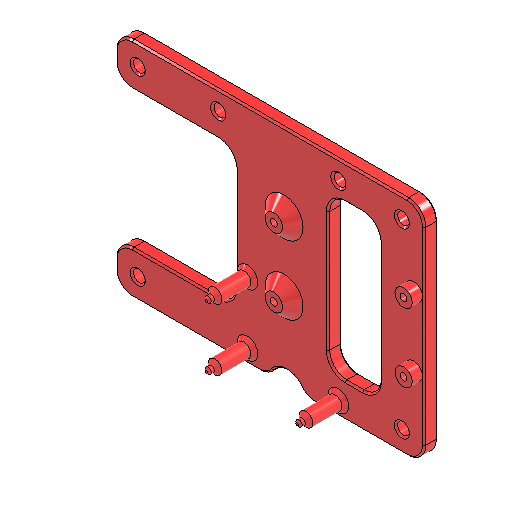
# Autodesk Inventor part: temp-logger-shelf
Saved by Autodesk Inventor 2026 (Build 300175050, 175E)
## iProperties
Created: 2025-07-16
Part Number: temp-logger-shelf
Material: ABS Plastic
Document SubType Name: Modeling
Designer: kuzmin
Density: 1.06 g/cm^3
Appearance: Light Red
Author: kuzmin
Autodesk Inventor part; units mm, degrees
ref_plane "YZ Plane" through (0, 0, 0) normal (1, 0, 0) x (0, 1, 0)
ref_plane "XZ Plane" through (0, 0, 0) normal (0, 1, 0) x (-1, 0, 0)
ref_plane "XY Plane" through (0, 0, 0) normal (0, 0, 1) x (1, 0, 0)
sketch "Sketch1" plane through (0, 0, 0) normal (0, 0, 1) x (1, 0, 0)
  line L0 (-45, 32.5) -> (45, 32.5)
  line L1 (45, 32.5) -> (45, -32.5)
  line L2 (45, -32.5) -> (-45, -32.5)
  line L3 (-45, -32.5) -> (-45, 32.5)
  line L4 (-38.5, 26.5) -> (38.5, 26.5) construction
  line L5 (38.5, 26.5) -> (38.5, -26.5) construction
  line L6 (38.5, -26.5) -> (-38.5, -26.5) construction
  line L7 (-38.5, -26.5) -> (-38.5, 26.5) construction
  circle A0 centre (-38.5, 26.5) radius 2
  circle A1 centre (38.5, 26.5) radius 2
  circle A2 centre (38.5, -26.5) radius 2
  circle A3 centre (-38.5, -26.5) radius 2
  point P0 (0, 0)
  point P1 (45, 0)
  point P2 (0, 32.5)
  point P3 (38.5, 0)
  point P4 (0, 26.5)
  dimension "d0" = 90
  dimension "d1" = 65
  dimension "d2" = 77
  dimension "d3" = 53
  dimension "d14" = 4
  constraints: 16 end point, 8 coincident, 4 centre point, 4 midpoint, 4 parallel, 3 equal radius, 2 horizontal, 2 horizontal alignment, 2 perpendicular, 2 vertical alignment
  measures "d0" distance of L0.start L0.end
  measures "d1" distance of L0.end L1.end
  measures "d2" distance of L4.start L4.end
  measures "d3" distance of L4.end L5.end
  measures "d14" diameter of A0
extrude "Extrusion1" add sketch "Sketch1" along normal blind 4 contours L0 L1 L2 L3 | A0 | A1 | A2 | A3
hole "Hole1" at (38.5, 26.5, 0) at (38.5, -26.5, 0) at (-38.5, -26.5, 0) at (-38.5, 26.5, 0) direction (0, 0, 1) diameter 3.4 end through all
sketch "Sketch2" plane through (0, 0, 4) normal (0, 0, 1) x (1, 0, 0)
  line L0 (-45, 20) -> (-10, 20)
  line L1 (-10, 20) -> (-10, -20)
  line L2 (-10, -20) -> (-45, -20)
  line L3 (-45, -20) -> (-45, 20)
  line L4 (-45, 32.5) -> (-45, -32.5) projected
  point P0 (0, 0)
  point P1 (-10, 0)
  dimension "d23" = 40
  dimension "d24" = 35
  constraints: 8 end point, 2 parallel, 1 horizontal, 1 horizontal alignment, 1 midpoint, 1 perpendicular, 1 point on line
  measures "d23" distance of L2.end L0.start
  measures "d24" distance of L0.start L0.end
extrude "Extrusion3" cut sketch "Sketch2" against normal blind 10
sketch "Sketch3" plane through (0, 0, 0) normal (0, 0, -1) x (-1, 0, 0)
  line L0 (-42, 10) -> (-4.2, 10) construction
  line L1 (-4.2, 10) -> (-4.2, -10) construction
  line L2 (-4.2, -10) -> (-42, -10) construction
  line L3 (-42, -10) -> (-42, 10) construction
  circle A0 centre (-42, 10) radius 2.5
  circle A1 centre (-4.2, 10) radius 2.5
  circle A2 centre (-4.2, -10) radius 2.5
  circle A3 centre (-42, -10) radius 2.5
  line L4 (-40, -32.5) -> (40, -32.5) projected
  line L5 (-45, -32.5) -> (-45, 32.5) projected
  point P0 (0, 0)
  point P1 (-4.2, 0)
  point P2 (-45, -27.5)
  point P3 (-45, 27.5)
  dimension "d27" = 20
  dimension "d28" = 37.8
  dimension "d30" = 5
  dimension "d47" = 3
  constraints: 8 coincident, 8 end point, 4 centre point, 3 equal radius, 2 parallel, 1 horizontal, 1 horizontal alignment, 1 midpoint, 1 perpendicular
  measures "d27" distance of L0.end L1.end
  measures "d28" distance of L0.start L0.end
  measures "d30" diameter of A1
  measures "d47" distance between parallel lines of L5 L3
extrude "Extrusion4" add sketch "Sketch3" against normal blind 7
hole "Hole2" at (4.2, 10, 0) at (4.2, -10, 0) at (42, -10, 0) at (42, 10, 0) direction (0, 0, 1) diameter 2 end through all
chamfer "Chamfer3" distance 3 angle 45 2 edges at (6.7, 10, 4) (6.7, -10, 4)
sketch "Sketch4" plane through (0, 0, 4) normal (0, 0, 1) x (1, 0, 0)
  line L0 (17, -22.5) -> (32, -22.5)
  line L1 (32, -22.5) -> (32, 22.5)
  line L2 (32, 22.5) -> (17, 22.5)
  line L3 (17, 22.5) -> (17, -22.5)
  line L4 (45, -32.5) -> (45, 32.5) projected
  line L5 (-45, -32.5) -> (45, -32.5) projected
  line L6 (0, -32.5) -> (10, -32.5)
  line L7 (10, -32.5) -> (10, -28.5)
  line L8 (10, -28.5) -> (0, -28.5)
  line L9 (0, -28.5) -> (0, -32.5)
  line L10 (-10, 20) -> (-10, -20) projected
  point P0 (0, 0)
  point P1 (17, 0)
  point P2 (45, -27.5)
  point P3 (45, 27.5)
  point P4 (-40, -32.5)
  point P5 (40, -32.5)
  point P6 (-10, 15)
  point P7 (-10, -15)
  dimension "d48" = 15
  dimension "d49" = 13
  dimension "d50" = 45
  dimension "d51" = 10
  dimension "d52" = 10
  dimension "d53" = 4
  constraints: 16 end point, 4 parallel, 2 horizontal, 2 midpoint, 2 perpendicular, 1 horizontal alignment
  measures "d48" distance of L1.end L2.end
  measures "d49" distance between parallel lines of L4 L1
  measures "d50" distance of L2.end L0.start
  measures "d51" distance between parallel lines of L10 L9
  measures "d52" distance of L7.end L8.end
  measures "d53" distance of L6.end L7.end
extrude "Extrusion5" cut sketch "Sketch4" against normal through all
fillet "Fillet2" radius 5 16 edges at (-10, -20, 2) (-10, 20, 2) (-45, 20, 2) (-45, 32.5, 2) (-45, -20, 2) (-45, -32.5, 2) (0, -28.5, 2) (0, -32.5, 2) (10, -28.5, 2) (10, -32.5, 2) (17, 22.5, 2) (32, 22.5, 2) (17, -22.5, 2) (32, -22.5, 2) (45, -32.5, 2) (45, 32.5, 2)
chamfer "Chamfer5" distance 0.5 angle 45 66 edges at (-21.5505, -32.5, 4) (26.5505, -32.5, 4) (-0.865, -31.9721, 4) (-43.5355, -31.0355, 4) (43.5355, -31.0355, 4) (10.865, -31.9721, 4) (7.3371, -29.0279, 4) (2.6629, -29.0279, 4) (-43.5355, -21.4645, 4) (-11.4645, -18.5355, 4) (-11.4645, 18.5355, 4) (-43.5355, 21.4645, 4) (-43.5355, 31.0355, 4) (43.5355, 31.0355, 4) (18.4645, -21.0355, 4) (30.5355, -21.0355, 4) (18.4645, 21.0355, 4) (30.5355, 21.0355, 4) (45, 0, 4) (0, 32.5, 4) (-45, -26.25, 4) (-45, 26.25, 4) (-27.5, 20, 4) (-10, 0, 4) (-27.5, -20, 4) (43.5355, 31.0355, 0) (0, 32.5, 0) (-43.5355, 31.0355, 0) (-45, -26.25, 0) (-45, 26.25, 0) (-43.5355, 21.4645, 0) (-27.5, 20, 0) (-11.4645, 18.5355, 0) (-10, 0, 0) (-11.4645, -18.5355, 0) (-27.5, -20, 0) (-43.5355, -21.4645, 0) (-43.5355, -31.0355, 0) (-21.5505, -32.5, 0) (26.5505, -32.5, 0) (-0.865, -31.9721, 0) (43.5355, -31.0355, 0) (10.865, -31.9721, 0) (7.3371, -29.0279, 0) (2.6629, -29.0279, 0) (18.4645, -21.0355, 0) (30.5355, -21.0355, 0) (18.4645, 21.0355, 0) (30.5355, 21.0355, 0) (45, 0, 0) (32, 0, 0) (24.5, -22.5, 0) (17, 0, 0) (24.5, 22.5, 0) (17, 0, 4) (24.5, 22.5, 4) (32, 0, 4) (24.5, -22.5, 4) (-38.5, 24.8, 4) (-38.5, -28.2, 4) (38.5, -28.2, 4) (38.5, 24.8, 4) (-38.5, 24.8, 0) (38.5, 24.8, 0) (38.5, -28.2, 0) (-38.5, -28.2, 0)
sketch "Sketch5" plane through (0, 0, 4) normal (0, 0, 1) x (1, 0, 0)
  line L0 (-45, 27.5) -> (-45, 25) projected
  line L1 (40, 32.5) -> (-40, 32.5) projected
  line L2 (-15, 27) -> (20, 27) construction
  point P0 (0, 0)
  dimension "d60" = 30
  dimension "d61" = 5.5
  dimension "d89" = 65
  constraints: 2 end point, 1 coincident, 1 horizontal
  measures "d60" distance from line of L0 L2.start
  measures "d61" distance from line of L1 L2.start
  measures "d89" distance from line of L0 L2.end
hole "Hole3" at (-15, 27, 4) at (20, 27, 4) direction (0, 0, -1) diameter 3.4 end through all
chamfer "Chamfer6" distance 0.5 angle 45 4 edges at (-15, 28.7, 4) (20, 28.7, 4) (20, 28.7, 0) (-15, 28.7, 0)
sketch "Sketch6" plane through (0, 0, 4) normal (0, 0, 1) x (1, 0, 0)
  line L0 (-6.5, -10.5) -> (20, -10.5) construction
  line L1 (20, -10.5) -> (20, -28.5) construction
  line L2 (20, -28.5) -> (-6.5, -28.5) construction
  line L3 (-6.5, -28.5) -> (-6.5, -10.5) construction
  line L4 (-10, 15) -> (-10, -15) projected
  line L5 (-40, -32.5) -> (-3.101, -32.5) projected
  circle A0 centre (-6.5, -10.5) radius 2
  circle A1 centre (-6.5, -28.5) radius 2
  circle A2 centre (20, -28.5) radius 2
  circle A3 centre (-6.5, -10.5) radius 0.9
  circle A4 centre (-6.5, -28.5) radius 0.9
  circle A5 centre (20, -28.5) radius 0.9
  point P0 (0, 0)
  dimension "d73" = 18
  dimension "d74" = 26.5
  dimension "d75" = 3.5
  dimension "d76" = 4
  dimension "d77" = 4
  dimension "d80" = 1.8
  constraints: 9 coincident, 8 end point, 6 centre point, 4 equal radius, 2 parallel, 1 horizontal, 1 perpendicular
  measures "d73" distance of L2.end L0.start
  measures "d74" distance of L0.start L0.end
  measures "d75" distance between parallel lines of L4 L3
  measures "d76" distance between parallel lines of L5 L2
  measures "d77" diameter of A2
  measures "d80" diameter of A3
extrude "Extrusion6" add sketch "Sketch6" along normal blind 10 contours A0 | A1 | A2 | A3 | A4 | A5
extrude "Extrusion7" add sketch "Sketch6" along normal blind 12 contours A3 | A4 | A5
chamfer "Chamfer7" distance 1 angle 45 3 edges at (-8.5, -28.5, 4) (18, -28.5, 4) (-8.5, -10.5, 4)
chamfer "Chamfer8" distance 0.55 angle 45 9 edges at (-8.5, -28.5, 14) (18, -28.5, 14) (-8.5, -10.5, 14) (-7.4, -10.5, 14) (-7.4, -28.5, 14) (19.1, -28.5, 14) (19.1, -28.5, 16) (-7.4, -10.5, 16) (-7.4, -28.5, 16)
equation "\"d4\" = thickness"
equation "\"d31\" = thickness + bump"
equation "\"thickness\" = 4"
equation "\"bump\" = 3"
body "Solid1"
